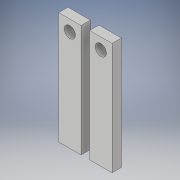
# Autodesk Inventor part: LC_sample_holder_clamp
Saved by Autodesk Inventor 2019 (Build 230136000, 136)
## iProperties
Created: 2021-05-27
Part Number: LC_sample_holder_clamp
Material: Generic
Document SubType Name: Modeling
Designer: marsikovabarbora
Density: 1 g/cm^3
Appearance: Default
Author: marsikovabarbora
Autodesk Inventor part; units mm, degrees
ref_plane "YZ Plane" through (0, 0, 0) normal (1, 0, 0) x (0, 1, 0)
ref_plane "XZ Plane" through (0, 0, 0) normal (0, 1, 0) x (-1, 0, 0)
ref_plane "XY Plane" through (0, 0, 0) normal (0, 0, 1) x (1, 0, 0)
sketch "Sketch1" plane through (0, 0, 0) normal (0, 0, 1) x (1, 0, 0)
  line L0 (-10.0097, 0) -> (10.0097, 0) construction
  line L1 (0, -21) -> (0, 21) construction
  line L2 (-7.1498, 15) -> (-1.1498, 15)
  line L3 (-1.1498, 15) -> (-1.1498, -15)
  line L4 (-1.1498, -15) -> (-7.1498, -15)
  line L5 (-7.1498, -15) -> (-7.1498, 15)
  circle A0 centre (-4.1498, 12) radius 1.5
  line L6 (-4.1498, 15) -> (-4.1498, -15) construction
  line L7 (7.1498, 15) -> (1.1498, 15)
  line L8 (1.1498, 15) -> (1.1498, -15)
  line L9 (1.1498, -15) -> (7.1498, -15)
  line L10 (7.1498, -15) -> (7.1498, 15)
  circle A1 centre (4.1498, 12) radius 1.5
  line L11 (4.1498, 15) -> (4.1498, -15) construction
  point P0 (0, 0)
  dimension "d0" = 6
  dimension "d1" = 3
  dimension "d2" = 3
  dimension "d3" = 30
  constraints: 20 end point, 8 symmetric about line, 4 midpoint, 4 point on line, 2 centre point, 2 parallel, 1 horizontal, 1 perpendicular, 2 other
  measures "d0" distance of L2.start L2.end
  measures "d1" diameter of A0
  measures "d2" distance from line of L2 A0.centre
  measures "d3" distance of L4.end L2.start
extrude "Extrusion1" add sketch "Sketch1" along normal blind 2.5
body "Solid1"
